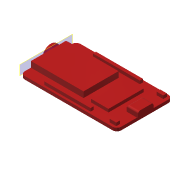
# Autodesk Inventor part: 00_ESP32_Board
Saved by Autodesk Inventor 2019 (Build 230136000, 136)
## iProperties
Created: 2021-09-09
Part Number: 00_ESP32_Board
Material: Generisch
Document SubType Name: Modeling
Designer: Muriel
Density: 1 g/cm^3
Appearance: Hellrot
Author: Muriel
Autodesk Inventor part; units mm, degrees
ref_plane "YZ Plane" through (0, 0, 0) normal (1, 0, 0) x (0, 1, 0)
ref_plane "XZ Plane" through (0, 0, 0) normal (0, 1, 0) x (-1, 0, 0)
ref_plane "XY Plane" through (0, 0, 0) normal (0, 0, 1) x (1, 0, 0)
sketch "Skizze1" plane through (0, 0, 0) normal (0, 1, 0) x (-1, 0, 0)
  line L0 (-21.35, -13.5) -> (21.35, -13.5)
  line L1 (23.35, -11.5) -> (23.35, 11.5)
  line L2 (21.35, 13.5) -> (-21.35, 13.5)
  line L3 (-23.35, 11.5) -> (-23.35, -11.5)
  line L4 (-23.35, -13.5) -> (23.35, 13.5) construction
  line L5 (23.35, -13.5) -> (-23.35, 13.5) construction
  arc A0 (23.35, 11.5) -> (21.35, 13.5) centre (21.35, 11.5) ccw
  arc A1 (21.35, -13.5) -> (23.35, -11.5) centre (21.35, -11.5) ccw
  arc A2 (-23.35, -11.5) -> (-21.35, -13.5) centre (-21.35, -11.5) ccw
  arc A3 (-21.35, 13.5) -> (-23.35, 11.5) centre (-21.35, 11.5) ccw
  point P0 (0, 0)
  dimension "d0" = 46.7
  dimension "d1" = 27
  dimension "d2" = 2
  constraints: 12 end point, 8 point on circle, 8 point on line, 8 tangent, 4 centre point, 3 equal radius, 2 midpoint, 2 parallel, 1 horizontal, 1 perpendicular
  measures "d0" distance of L5.end L4.end
  measures "d1" distance of L4.end L5.start
  measures "d2" radius of A0
extrude "Extrusion1" add sketch "Skizze1" along normal blind 1.5
sketch "Skizze2" plane through (0, 1.5, 0) normal (0, 1, 0) x (1, 0, 0)
  line L0 (-21.35, -13.5) -> (21.35, -13.5) projected
  arc A0 (21.35, -13.5) -> (23.35, -11.5) centre (21.35, -11.5) ccw projected
  line L1 (23.35, -11.5) -> (23.35, 11.5) projected
  arc A1 (23.35, 11.5) -> (21.35, 13.5) centre (21.35, 11.5) ccw projected
  line L2 (21.35, 13.5) -> (-21.35, 13.5) projected
  arc A2 (-21.35, 13.5) -> (-23.35, 11.5) centre (-21.35, 11.5) ccw projected
  line L3 (-23.35, 11.5) -> (-23.35, -11.5) projected
  arc A3 (-23.35, -11.5) -> (-21.35, -13.5) centre (-21.35, -11.5) ccw projected
  line L4 (18.35, -3.75) -> (23.85, -3.75)
  line L5 (23.85, -3.75) -> (23.85, 3.75)
  line L6 (23.85, 3.75) -> (18.35, 3.75)
  line L7 (18.35, 3.75) -> (18.35, -3.75)
  line L8 (18.35, -3.75) -> (23.85, 3.75) construction
  line L9 (23.85, -3.75) -> (18.35, 3.75) construction
  point P0 (0, 0)
  point P1 (21.1, 0)
  dimension "d5" = 5.5
  dimension "d6" = 7.5
  dimension "d7" = 0.5
  constraints: 12 end point, 2 midpoint, 2 parallel, 1 horizontal, 1 perpendicular
  measures "d5" distance of L6.end L5.end
  measures "d6" distance of L5.end L4.end
  measures "d7" distance between parallel lines of L5 L1
extrude "Extrusion2" add sketch "Skizze2" along normal blind 2.8 contours L4 L7 L6 L1 | L1 L6 L5 L4
fillet "Rundung1" radius 1 3 edges at (21.1, 4.3, 3.75) (21.1, 4.3, -3.75) (18.35, 4.3, 0)
sketch "Skizze3" plane through (0, 1.5, 0) normal (0, -1, 0) x (1, 0, 0)
  line L0 (-21.35, 13.5) -> (21.35, 13.5) projected
  arc A0 (-21.35, 13.5) -> (-23.35, 11.5) centre (-21.35, 11.5) ccw projected
  line L1 (-23.35, -11.5) -> (-23.35, 11.5) projected
  arc A1 (-23.35, -11.5) -> (-21.35, -13.5) centre (-21.35, -11.5) ccw projected
  line L2 (21.35, -13.5) -> (-21.35, -13.5) projected
  arc A2 (21.35, -13.5) -> (23.35, -11.5) centre (21.35, -11.5) ccw projected
  line L3 (23.35, 11.5) -> (23.35, -11.5) projected
  arc A3 (23.35, 11.5) -> (21.35, 13.5) centre (21.35, 11.5) ccw projected
  line L4 (2.15, -8.5) -> (-23.35, -8.5)
  line L5 (-23.35, -8.5) -> (-23.35, 8.5)
  line L6 (-23.35, 8.5) -> (2.15, 8.5)
  line L7 (2.15, 8.5) -> (2.15, -8.5)
  line L8 (2.15, -8.5) -> (-23.35, 8.5) construction
  line L9 (-23.35, -8.5) -> (2.15, 8.5) construction
  point P0 (0, 0)
  point P1 (-10.6, 0)
  point P2 (-23.35, 0)
  dimension "d11" = 25.5
  dimension "d12" = 17
  constraints: 12 end point, 4 midpoint, 2 parallel, 1 horizontal, 1 perpendicular
  measures "d11" distance of L5.end L6.end
  measures "d12" distance of L4.end L5.end
extrude "Extrusion3" add sketch "Skizze3" against normal blind 2.8 contours L6 L7 L4 L1
sketch "Skizze5" plane through (0, 0, 0) normal (0, -1, 0) x (1, 0, 0)
  line L0 (-21.35, 13.5) -> (21.35, 13.5) projected
  arc A0 (-21.35, 13.5) -> (-23.35, 11.5) centre (-21.35, 11.5) ccw projected
  line L1 (-23.35, -11.5) -> (-23.35, 11.5) projected
  arc A1 (-23.35, -11.5) -> (-21.35, -13.5) centre (-21.35, -11.5) ccw projected
  line L2 (21.35, -13.5) -> (-21.35, -13.5) projected
  arc A2 (21.35, -13.5) -> (23.35, -11.5) centre (21.35, -11.5) ccw projected
  line L3 (23.35, 11.5) -> (23.35, -11.5) projected
  arc A3 (23.35, 11.5) -> (21.35, 13.5) centre (21.35, 11.5) ccw projected
  line L4 (-5.5686, -8.25) -> (-10.35, -8.25)
  line L5 (-10.35, -8.25) -> (-10.35, 8.25)
  line L6 (-10.35, 8.25) -> (-5.5686, 8.25)
  line L7 (-5.5686, 8.25) -> (-5.5686, -8.25)
  line L8 (-5.5686, -8.25) -> (-10.35, 8.25) construction
  line L9 (-10.35, -8.25) -> (-5.5686, 8.25) construction
  line L10 (15.35, -7.5) -> (0.35, -7.5)
  line L11 (0.35, -7.5) -> (0.35, 7.5)
  line L12 (0.35, 7.5) -> (15.35, 7.5)
  line L13 (15.35, 7.5) -> (15.35, -7.5)
  line L14 (15.35, -7.5) -> (0.35, 7.5) construction
  line L15 (0.35, -7.5) -> (15.35, 7.5) construction
  point P0 (0, 0)
  point P1 (-7.9593, 0)
  point P2 (7.85, 0)
  dimension "d23" = 15
  dimension "d24" = 15
  dimension "d25" = 13
  dimension "d26" = 16.5
  dimension "d27" = 8
  constraints: 24 end point, 4 midpoint, 4 parallel, 2 horizontal, 2 perpendicular
  measures "d23" distance of L11.end L12.end
  measures "d24" distance of L10.end L11.end
  measures "d25" distance between parallel lines of L5 L1
  measures "d26" distance between parallel lines of L4 L6
  measures "d27" distance between parallel lines of L3 L13
extrude "Extrusion5" add sketch "Skizze5" along normal blind 2 contours L4 L5 L6 L7 | L10 L11 L12 L13
ref_plane "Arbeitsebene1" through (-24.35, 0, -11.5) normal (-1, 0, 0) x (0, 0, 1)
sketch "Skizze8" plane through (-24.35, 0, -11.5) normal (-1, 0, 0) x (0, 0, 1)
  line L0 (8, 0.6) -> (-1, 0.6)
  line L1 (-1, 0.6) -> (-1, -8.4)
  line L2 (-1, -8.4) -> (8, -8.4)
  line L3 (8, -8.4) -> (8, 0.6)
  line L4 (8, 0.6) -> (-1, -8.4) construction
  line L5 (-1, 0.6) -> (8, -8.4) construction
  line L6 (0, 0) -> (23, 0) projected
  line L7 (3, 4.3) -> (20, 4.3) projected
  line L8 (19.75, -2) -> (3.25, -2) projected
  line L9 (0, 0) -> (-2, 0) projected
  line L10 (-2, 0) -> (-2, 1.5) projected
  point P0 (11.5, 0)
  point P1 (3.5, -3.9)
  dimension "d40" = 9
  dimension "d41" = 9
  dimension "d54" = 1
  dimension "d62" = 0.6
  constraints: 12 end point, 2 midpoint, 2 parallel, 1 horizontal, 1 perpendicular
  measures "d40" distance of L2.end L1.end
  measures "d41" distance of L1.end L0.end
  measures "d54" distance between parallel lines of L1 L10
  measures "d62" distance between parallel lines of L0 L6
extrude "Extrusion8" add sketch "Skizze8" along normal blind 2.1
sketch "Skizze9" plane through (-26.45, 0, -11.5) normal (-1, 0, 0) x (0, 0, 1)
  line L0 (8, 0.6) -> (-1, 0.6) projected
  line L1 (-1, 0.6) -> (-1, -8.4) projected
  line L2 (-1, -8.4) -> (8, -8.4) projected
  line L3 (8, -8.4) -> (8, 0.6) projected
  circle A0 centre (3.5, -3.9) radius 4
  point P0 (11.5, 0)
  dimension "d45" = 8
  dimension "d49" = 4.5
  dimension "d50" = 4.5
  constraints: 1 centre point
  measures "d45" diameter of A0
  measures "d49" distance from line of A0.centre L0
  measures "d50" distance from line of L3 A0.centre
extrude "Extrusion9" add sketch "Skizze9" along normal blind 3.8 contours A0
sketch "Skizze10" plane through (0, 1.5, 0) normal (0, 1, 0) x (1, 0, 0)
  line L0 (2.15, -8.5) -> (-23.35, -8.5) projected
  line L1 (-23.35, -8.5) -> (-23.35, -11.5) projected
  arc A0 (-23.35, -11.5) -> (-21.35, -13.5) centre (-21.35, -11.5) ccw projected
  line L2 (-21.35, -13.5) -> (21.35, -13.5) projected
  arc A1 (21.35, -13.5) -> (23.35, -11.5) centre (21.35, -11.5) ccw projected
  line L3 (23.35, -11.5) -> (23.35, -3.75) projected
  line L4 (23.35, -3.75) -> (18.35, -3.75) projected
  line L5 (18.35, -3.75) -> (18.35, 3.75) projected
  line L6 (18.35, 3.75) -> (23.35, 3.75) projected
  line L7 (23.35, 3.75) -> (23.35, 11.5) projected
  arc A2 (23.35, 11.5) -> (21.35, 13.5) centre (21.35, 11.5) ccw projected
  line L8 (21.35, 13.5) -> (-21.35, 13.5) projected
  arc A3 (-21.35, 13.5) -> (-23.35, 11.5) centre (-21.35, 11.5) ccw projected
  line L9 (-23.35, 11.5) -> (-23.35, 8.5) projected
  line L10 (-23.35, 8.5) -> (2.15, 8.5) projected
  line L11 (2.15, 8.5) -> (2.15, -8.5) projected
  line L12 (21.893, 12.205) -> (18.6612, 12.205)
  line L13 (18.6612, 12.205) -> (18.6612, 10.419)
  line L14 (18.6612, 10.419) -> (21.893, 10.419)
  line L15 (21.893, 10.419) -> (21.893, 12.205)
  line L16 (21.893, -10.5027) -> (18.6612, -10.5027)
  line L17 (18.6612, -10.5027) -> (18.6612, -12.3737)
  line L18 (18.6612, -12.3737) -> (21.893, -12.3737)
  line L19 (21.893, -12.3737) -> (21.893, -10.5027)
  line L20 (14.2522, 8.5) -> (5.7379, 8.5)
  line L21 (5.7379, 8.5) -> (5.7379, -8.5)
  line L22 (5.7379, -8.5) -> (14.2522, -8.5)
  line L23 (14.2522, -8.5) -> (14.2522, 8.5)
  line L24 (9.5652, -12.5) -> (-12.7904, -12.5)
  line L25 (-12.7904, -12.5) -> (-12.7904, -11)
  line L26 (-12.7904, -11) -> (9.5652, -11)
  line L27 (9.5652, -11) -> (9.5652, -12.5)
  line L28 (9.995, 11) -> (-12.7904, 11)
  line L29 (-12.7904, 11) -> (-12.7904, 12.5)
  line L30 (-12.7904, 12.5) -> (9.995, 12.5)
  line L31 (9.995, 12.5) -> (9.995, 11)
  point P0 (0, 0)
  dimension "d58" = 1
  dimension "d59" = 1
  dimension "d60" = 1.5
  dimension "d61" = 1.5
  constraints: 40 end point, 10 parallel, 5 horizontal, 5 perpendicular, 3 point on line
  measures "d58" distance between parallel lines of L30 L8
  measures "d59" distance between parallel lines of L2 L24
  measures "d60" distance between parallel lines of L30 L28
  measures "d61" distance between parallel lines of L26 L24
extrude "Extrusion10" add sketch "Skizze10" along normal blind 1.5 contours L15 L14 L13 L12 | L19 L18 L17 L16 | L23 L22 L21 L20 | L24 L25 L26 L27 | L28 L29 L30 L31
